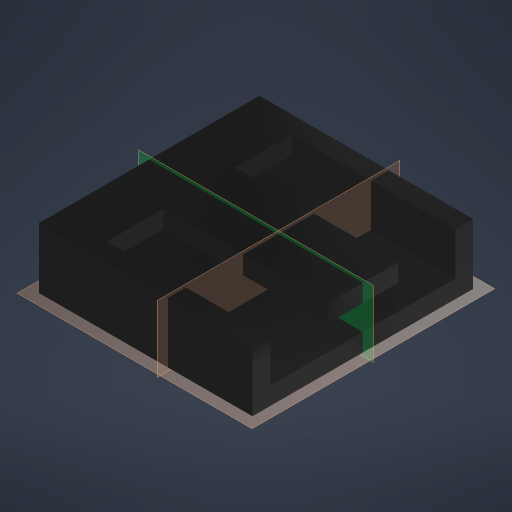
# Autodesk Inventor part: LOLIN C3 Mini Holder
Saved by Autodesk Inventor 2024 (Build 280153000, 153)
## iProperties
Manager: Louis Van Roosmaelen
Company: DCS - DIGITAL COMBAT SIMULATOR
Created: 2023-11-01
Part Number: LOLIN C3 Mini Holder
Material: S235
Catalog Web Link: http://emmausbovenbouw.op-weg.be/
Vendor: Emmaüsinstituut Bovenbouw Aalter
Document SubType Name: Modeling
Designer: Louis
Engineer: Declercq St.
Manufacturer: Standard
Standards Organization: Custom
Density: 7.86 g/cm^3
Appearance: Smooth - Black
IDENT.NR.: AJ2022
TEAM: 30
Title: F18C Home Cockpit
Author: Louis
Keywords: Ø
Autodesk Inventor part; units mm, degrees
sketch "Sketch1" plane through (0, 0, 0) normal (0, 0, 1) x (1, 0, 0)
  line L0 (0, 2.8582) -> (0, -2.8582) construction
  line L1 (-5.7775, 0) -> (5.7775, 0) construction
  line L2 (-18.15, -15.5) -> (18.15, -15.5)
  line L3 (18.15, -15.5) -> (18.15, 15.5)
  line L4 (18.15, 15.5) -> (-18.15, 15.5)
  line L5 (-18.15, 15.5) -> (-18.15, -15.5)
  line L6 (-18.15, -15.5) -> (18.15, 15.5) construction
  line L7 (18.15, -15.5) -> (-18.15, 15.5) construction
  point P0 (0, 0)
  point P1 (0, 0)
  dimension "d0" = 36.3
  dimension "d1" = 31
  constraints: 16 end point, 4 midpoint, 2 horizontal, 2 parallel, 1 coincident, 1 perpendicular, 1 vertical
  measures "d0" distance of L4.end L3.end
  measures "d1" distance of L3.end L2.end
extrude "Extrusion1" add sketch "Sketch1" along normal blind 2.5
sketch "Sketch2" plane through (0, 0, 2.5) normal (0, 0, 1) x (1, 0, 0)
  line L0 (18.15, -15.5) -> (-18.15, -15.5) projected
  line L1 (-18.15, -15.5) -> (-18.15, 15.5) projected
  line L2 (-18.15, 15.5) -> (18.15, 15.5) projected
  line L3 (18.15, 15.5) -> (18.15, -15.5) projected
  line L4 (-18.15, 15.5) -> (-16.15, 15.5)
  line L5 (-16.15, 15.5) -> (-16.15, -15.5)
  line L6 (-16.15, -15.5) -> (-18.15, -15.5)
  line L7 (-18.15, -15.5) -> (-18.15, 15.5)
  point P0 (0, 0)
  dimension "d4" = 2
  constraints: 8 end point, 2 parallel, 1 horizontal, 1 perpendicular, 1 point on line
  measures "d4" distance of L5.end L6.end
extrude "Extrusion2" add sketch "Sketch2" along normal blind 3.5 contours L0 L1 L2 L5
sketch "Sketch3" plane through (0, 0, 6) normal (0, 0, 1) x (1, 0, 0)
  line L0 (-16.15, 15.5) -> (-16.15, -15.5) projected
  line L1 (-16.15, -15.5) -> (-18.15, -15.5) projected
  line L2 (-18.15, -15.5) -> (-18.15, 15.5) projected
  line L3 (-18.15, 15.5) -> (-16.15, 15.5) projected
  line L4 (-18.15, 5) -> (11.85, 5)
  line L5 (11.85, 5) -> (11.85, -5)
  line L6 (11.85, -5) -> (-18.15, -5)
  line L7 (-18.15, -5) -> (-18.15, 5)
  line L8 (-25.41, 0) -> (25.41, 0) projected
  point P0 (0, 0)
  point P1 (-16.15, 5)
  point P2 (-16.15, -5)
  dimension "d7" = 10
  dimension "d8" = 5
  dimension "d9" = 30
  constraints: 8 end point, 2 parallel, 1 horizontal, 1 perpendicular, 1 point on line
  measures "d7" distance of L4.end L5.end
  measures "d8" distance between parallel lines of L8 L4
  measures "d9" distance of L5.end L6.end
extrude "Extrusion3" add sketch "Sketch3" along normal blind 2.5
sketch "Sketch4" plane through (0, 0, 2.5) normal (0, 0, 1) x (1, 0, 0)
  line L0 (-16.15, 15.5) -> (-16.15, -15.5) projected
  line L1 (18.15, -15.5) -> (-16.15, -15.5) projected
  line L2 (18.15, 15.5) -> (18.15, -15.5) projected
  line L3 (-16.15, 15.5) -> (18.15, 15.5) projected
  line L4 (-18.15, 15.5) -> (-16.15, 15.5) projected
  line L5 (-18.15, -15.5) -> (-18.15, 15.5) projected
  line L6 (-16.15, -15.5) -> (-18.15, -15.5) projected
  line L7 (-16.15, 15.5) -> (11.85, 15.5)
  line L8 (11.85, 15.5) -> (11.85, 13)
  line L9 (11.85, 13) -> (-16.15, 13)
  line L10 (-16.15, 13) -> (-16.15, 15.5)
  line L11 (-16.15, -15.5) -> (11.85, -15.5)
  line L12 (11.85, -15.5) -> (11.85, -13)
  line L13 (11.85, -13) -> (-16.15, -13)
  line L14 (-16.15, -13) -> (-16.15, -15.5)
  point P0 (18.15, 13.5)
  point P1 (11.85, -15.5)
  point P2 (11.85, 15.5)
  dimension "d16" = 2.5
  dimension "d17" = 6.3
  dimension "d18" = 6.3
  dimension "d19" = 2.5
  constraints: 16 end point, 4 parallel, 2 horizontal, 2 perpendicular, 1 point on line
  measures "d16" distance of L7.end L8.end
  measures "d17" distance between parallel lines of L2 L8
  measures "d18" distance between parallel lines of L2 L12
  measures "d19" distance between parallel lines of L1 L13
extrude "Extrusion4" add sketch "Sketch4" along normal up to surface (6 mm away) contours L3 L8 L9 L0 | L13 L12 L1 L0
sketch "Sketch5" plane through (0, 0, 2.5) normal (0, 0, 1) x (1, 0, 0)
  line L0 (11.85, 13) -> (-16.15, 13) projected
  line L1 (-16.15, -13) -> (-16.15, 13) projected
  line L2 (-16.15, -13) -> (11.85, -13) projected
  line L3 (11.85, -13) -> (11.85, -15.5) projected
  line L4 (18.15, -15.5) -> (11.85, -15.5) projected
  line L5 (18.15, 15.5) -> (18.15, -15.5) projected
  line L6 (11.85, 15.5) -> (18.15, 15.5) projected
  line L7 (11.85, 15.5) -> (11.85, 13) projected
  line L8 (11.85, -15.5) -> (-18.15, -15.5) projected
  line L9 (-18.15, -15.5) -> (-18.15, 15.5) projected
  line L10 (-18.15, 15.5) -> (11.85, 15.5) projected
  line L11 (18.15, -15.5) -> (11.85, -15.5)
  line L12 (11.85, -15.5) -> (11.85, 15.5)
  line L13 (11.85, 15.5) -> (18.15, 15.5)
  line L14 (18.15, 15.5) -> (18.15, -15.5)
  point P0 (0, 0)
  constraints: 8 end point, 2 parallel, 1 horizontal, 1 perpendicular
extrude "Extrusion5" cut sketch "Sketch5" against normal up to surface (2.5 mm away) contours L7 L6 L5 L4 L3 L12
sketch "Sketch6" plane through (-16.15, -5, 6) normal (1, 0, 0) x (0, 0, -1)
  line L0 (0, 0) -> (-2.5, 0) projected
  line L1 (-2.5, -8) -> (-2.5, 0) projected
  line L2 (-2.5, -10.5) -> (-2.5, -8) projected
  line L3 (6, -10.5) -> (-2.5, -10.5) projected
  line L4 (6, 20.5) -> (6, -10.5) projected
  line L5 (-2.5, 20.5) -> (6, 20.5) projected
  line L6 (-2.5, 18) -> (-2.5, 20.5) projected
  line L7 (-2.5, 10) -> (-2.5, 18) projected
  line L8 (-2.5, 0) -> (-2.5, 10) projected
  line L9 (0, 10) -> (0, 0) projected
  line L10 (-2.5, 10) -> (0, 10) projected
  line L11 (-2.5, -8) -> (3.5, -8) projected
  line L12 (3.5, -8) -> (3.5, 18) projected
  line L13 (3.5, 18) -> (-2.5, 18) projected
  line L14 (0, 0) -> (-2.5, 0)
  line L15 (-2.5, 0) -> (-2.5, -8)
  line L16 (-2.5, -8) -> (0, -8)
  line L17 (0, -8) -> (0, 0)
  line L18 (-2.5, 10) -> (-2.5, 18) projected
  line L19 (0, 10) -> (-2.5, 10)
  line L20 (-2.5, 10) -> (-2.5, 18)
  line L21 (-2.5, 18) -> (0, 18)
  line L22 (0, 18) -> (0, 10)
  point P0 (6, 5)
  constraints: 16 end point, 4 parallel, 2 horizontal, 2 perpendicular
extrude "Extrusion6" add sketch "Sketch6" along normal blind 5 contours L17 L11 L1 L0 | L10 L7 L13 L22
equation "\"d8\" = 0.5 * d7"
equation "\"d18\" = d17"
equation "\"d19\" = d16"
body "Solid1"
